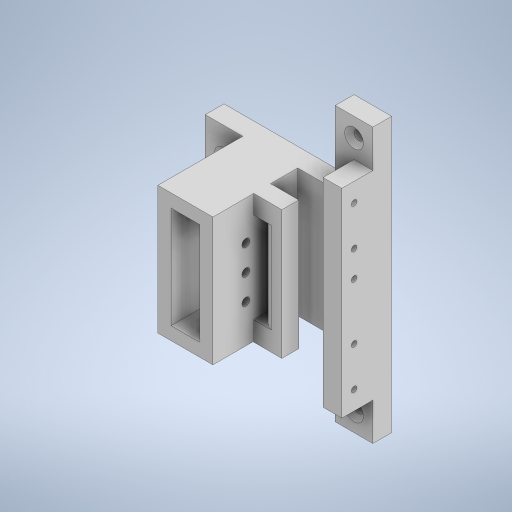
# Autodesk Inventor part: base
Saved by Autodesk Inventor 2024 (Build 280153000, 153)
## iProperties
Created: 2024-06-17
Part Number: base
Material: Generic
Document SubType Name: Modeling
Designer: omiye
Density: 1 g/cm^3
Appearance: Default
Author: omiye
Autodesk Inventor part; units mm, degrees
ref_plane "YZ Plane" through (0, 0, 0) normal (1, 0, 0) x (0, 1, 0)
ref_plane "XZ Plane" through (0, 0, 0) normal (0, 1, 0) x (-1, 0, 0)
ref_plane "XY Plane" through (0, 0, 0) normal (0, 0, 1) x (1, 0, 0)
sketch "Sketch1" plane through (0, 0, 0) normal (1, 0, 0) x (0, 1, 0)
  line L0 (27.1, -22.6) -> (-27.1, -22.6)
  line L1 (-27.1, -22.6) -> (-27.1, 22.6)
  line L2 (-27.1, 22.6) -> (27.1, 22.6)
  line L3 (27.1, 22.6) -> (27.1, -22.6)
  line L4 (27.1, -22.6) -> (-27.1, 22.6) construction
  line L5 (-27.1, -22.6) -> (27.1, 22.6) construction
  point P0 (0, 0)
  dimension "d0" = 54.2
  dimension "d1" = 45.2
  constraints: 12 end point, 2 midpoint, 2 parallel, 1 horizontal, 1 perpendicular
  measures "d0" distance of L1.end L2.end
  measures "d1" distance of L0.end L1.end
extrude "Extrusion1" add sketch "Sketch1" along normal blind 15.3
sketch "Sketch2" plane through (0, 27.1, 22.6) normal (0, 1, 0) x (1, 0, 0)
  line L0 (15.3, 0) -> (15.3, 45.2) projected
  line L1 (0, 0) -> (0, 45.2) projected
  line L2 (15.3, 0) -> (0, 0)
  line L3 (0, 0) -> (0, 45.2)
  line L4 (0, 45.2) -> (15.3, 45.2)
  line L5 (15.3, 45.2) -> (15.3, 0)
  point P0 (0, 22.6)
  constraints: 8 end point, 2 parallel, 1 horizontal, 1 perpendicular
extrude "Extrusion2" add sketch "Sketch2" along normal blind 7
sketch "Sketch3" plane through (0, -27.1, -22.6) normal (0, -1, 0) x (1, 0, 0)
  line L0 (0, 45.2) -> (0, 0) projected
  line L1 (15.3, 45.2) -> (15.3, 0) projected
  line L2 (0, 45.2) -> (15.3, 45.2)
  line L3 (15.3, 45.2) -> (15.3, 0)
  line L4 (15.3, 0) -> (0, 0)
  line L5 (0, 0) -> (0, 45.2)
  point P0 (0, 22.6)
  constraints: 8 end point, 2 parallel, 1 horizontal, 1 perpendicular
extrude "Extrusion3" add sketch "Sketch3" along normal blind 7
sketch "Sketch4" plane through (15.3, 0, 0) normal (1, 0, 0) x (0, 0, -1)
  line L0 (-22.6, -34.1) -> (-22.6, 34.1) projected
  line L1 (-22.6, 34.1) -> (22.6, 34.1) projected
  line L2 (-22.6, -34.1) -> (22.6, -34.1)
  line L3 (22.6, -34.1) -> (22.6, 34.1)
  line L4 (22.6, 34.1) -> (-22.6, 34.1)
  line L5 (-22.6, 34.1) -> (-22.6, -34.1)
  point P0 (0, 0)
  constraints: 8 end point, 2 parallel, 1 horizontal, 1 perpendicular
extrude "Extrusion4" add sketch "Sketch4" along normal blind 7
sketch "Sketch5" plane through (0, 0, 0) normal (-1, 0, 0) x (0, 0, 1)
  line L0 (-22.6, 34.1) -> (22.6, 34.1) projected
  line L1 (22.6, -34.1) -> (-22.6, -34.1) projected
  line L2 (22.6, 34.1) -> (-22.6, 34.1)
  line L3 (-22.6, 34.1) -> (-22.6, -34.1)
  line L4 (-22.6, -34.1) -> (22.6, -34.1)
  line L5 (22.6, -34.1) -> (22.6, 34.1)
  point P0 (0, 0)
  constraints: 8 end point, 2 parallel, 1 horizontal, 1 perpendicular
extrude "Extrusion5" add sketch "Sketch5" along normal blind 7
sketch "Sketch6" plane through (22.3, -34.1, -22.6) normal (0, 0, -1) x (-1, 0, 0)
  line L0 (29.3, 0) -> (0, 0) projected
  line L1 (0, 68.2) -> (0, 0) projected
  line L2 (29.3, 0) -> (0, 0)
  line L3 (0, 0) -> (0, 68.2)
  line L4 (0, 68.2) -> (29.3, 68.2)
  line L5 (29.3, 68.2) -> (29.3, 0)
  point P0 (22.3, 34.1)
  constraints: 8 end point, 2 parallel, 1 horizontal, 1 perpendicular
extrude "Extrusion6" add sketch "Sketch6" along normal blind 10
sketch "Sketch7" plane through (-7, 0, 0) normal (-1, 0, 0) x (0, 0, 1)
  line L0 (22.6, 34.1) -> (-32.6, 34.1) projected
  line L1 (22.6, -34.1) -> (-32.6, -34.1) projected
  line L2 (-32.6, 34.1) -> (-22.6, 34.1)
  line L3 (-22.6, 34.1) -> (-22.6, -34.1)
  line L4 (-22.6, -34.1) -> (-32.6, -34.1)
  line L5 (-32.6, -34.1) -> (-32.6, 34.1)
  point P0 (0, 0)
  dimension "d14" = 10
  constraints: 8 end point, 2 parallel, 1 horizontal, 1 perpendicular, 1 point on line
  measures "d14" distance of L3.end L4.end
extrude "Extrusion7" add sketch "Sketch7" along normal blind 20
sketch "Sketch8" plane through (22.3, -34.1, 22.6) normal (0, 0, 1) x (1, 0, 0)
  line L0 (0, 68.2) -> (-49.3, 68.2) projected
  line L1 (-29.3, 0) -> (-29.3, 68.2) projected
  line L2 (0, 68.2) -> (-29.3, 68.2)
  line L3 (-29.3, 68.2) -> (-29.3, 0)
  line L4 (-29.3, 0) -> (0, 0)
  line L5 (0, 0) -> (0, 68.2)
  line L6 (-22.25, 7) -> (-7.05, 7)
  line L7 (-7.05, 7) -> (-7.05, 61.2)
  line L8 (-7.05, 61.2) -> (-22.25, 61.2)
  line L9 (-22.25, 61.2) -> (-22.25, 7)
  line L10 (-22.25, 7) -> (-7.05, 61.2) construction
  line L11 (-7.05, 7) -> (-22.25, 61.2) construction
  point P0 (-22.3, 34.1)
  point P1 (-14.65, 34.1)
  dimension "d17" = 15.2
  dimension "d18" = 54.2
  constraints: 20 end point, 4 parallel, 2 horizontal, 2 midpoint, 2 perpendicular
  measures "d17" distance of L8.end L7.end
  measures "d18" distance of L7.end L6.end
extrude "Extrusion8" cut sketch "Sketch8" against normal blind 45.2 contours L9 L8 L7 L6
sketch "Sketch9" plane through (22.3, 0, 0) normal (1, 0, 0) x (0, 0, -1)
  line L0 (-22.6, -27.1) -> (22.6, -27.1) projected
  line L1 (-22.6, 27.1) -> (22.6, 27.1) projected
  line L2 (-22.6, -27.1) -> (22.6, -27.1)
  line L3 (22.6, -27.1) -> (22.6, 27.1)
  line L4 (22.6, 27.1) -> (-22.6, 27.1)
  line L5 (-22.6, 27.1) -> (-22.6, -27.1)
  line L6 (-22.6, -27.1) -> (-5.1, -27.1)
  circle A0 centre (-5.1, -13.7) radius 2.1
  circle A1 centre (-5.1, -0.2) radius 2.1
  circle A2 centre (-5.1, 13.4) radius 2.1
  circle A3 centre (12.4, -13.7) radius 2.1
  circle A4 centre (12.4, -0.2) radius 2.1
  circle A5 centre (12.4, 13.4) radius 2.1
  point P0 (0, 0)
  constraints: 10 end point, 6 centre point, 2 parallel, 1 horizontal, 1 perpendicular, 1 point on line
extrude "Extrusion9" cut sketch "Sketch9" against normal blind 39.25 contours A0 | A1 | A2 | A3 | A4 | A5
sketch "Sketch10" plane through (22.3, 0, 0) normal (1, 0, 0) x (0, 0, -1)
  line L0 (-22.6, -34.1) -> (32.6, -34.1) projected
  line L1 (-22.6, 34.1) -> (32.6, 34.1) projected
  line L2 (32.6, -34.1) -> (22.6, -34.1)
  line L3 (22.6, -34.1) -> (22.6, 34.1)
  line L4 (22.6, 34.1) -> (32.6, 34.1)
  line L5 (32.6, 34.1) -> (32.6, -34.1)
  point P0 (0, 0)
  dimension "d36" = 10
  constraints: 8 end point, 2 parallel, 1 horizontal, 1 perpendicular, 1 point on line
  measures "d36" distance of L3.end L4.end
extrude "Extrusion10" add sketch "Sketch10" along normal blind 20
sketch "Sketch11" plane through (42.3, 0, 0) normal (1, 0, 0) x (0, 0, -1)
  line L0 (32.6, 73) -> (22.6, 73)
  line L1 (22.6, 73) -> (22.6, -73)
  line L2 (22.6, -73) -> (32.6, -73)
  line L3 (32.6, -73) -> (32.6, 73)
  line L4 (32.6, 73) -> (22.6, -73) construction
  line L5 (22.6, 73) -> (32.6, -73) construction
  point P0 (0, 0)
  point P1 (27.6, 0)
  dimension "d62" = 10
  dimension "d63" = 146
  constraints: 12 end point, 2 midpoint, 2 parallel, 1 horizontal, 1 perpendicular
  measures "d62" distance of L2.end L1.end
  measures "d63" distance of L1.end L0.end
sketch "Sketch12" plane through (22.3, 0, 0) normal (1, 0, 0) x (0, 0, -1)
  circle A0 centre (-5.1, -0.2) radius 2.1 projected
  circle A1 centre (12.4, -0.2) radius 2.1 projected
  line L0 (-5.1, -0.2) -> (12.4, -0.2)
  line L1 (-22.6, 27.1) -> (22.6, 27.1) projected
  line L2 (-0.85, -27.5) -> (8.15, -27.5)
  line L3 (8.15, -27.5) -> (8.15, 27.1)
  line L4 (8.15, 27.1) -> (-0.85, 27.1)
  line L5 (-0.85, 27.1) -> (-0.85, -27.5)
  line L6 (-0.85, -27.5) -> (8.15, 27.1) construction
  line L7 (8.15, -27.5) -> (-0.85, 27.1) construction
  point P0 (0, 0)
  point P1 (3.65, -0.2)
  dimension "d42" = 9
  constraints: 14 end point, 3 midpoint, 2 horizontal, 2 parallel, 1 perpendicular, 1 point on line
  measures "d42" distance of L4.end L3.end
extrude "Extrusion12" add sketch "Sketch12" along normal blind 15 contours L5 L1 L3 L0 | L0 L3 L2 L5
sketch "Sketch13" plane through (22.3, -27.5, 0.85) normal (0, 0, 1) x (1, 0, 0)
  line L0 (0, 0) -> (15, 0) projected
  line L1 (15, 0) -> (15, 10)
  line L2 (15, 54.6) -> (15, 0) projected
  line L3 (15, 0) -> (25, 0) construction
  line L4 (0, 54.6) -> (15, 54.6) projected
  line L5 (15, 54.6) -> (15, 44.6)
  line L6 (0, 54.6) -> (0, 0) projected
  line L7 (5, 10) -> (5, 44.6)
  line L8 (0, 44.6) -> (0, 10)
  line L9 (0, -6.6) -> (0, 3.4)
  line L10 (0, 61.6) -> (0, 51.6)
  line L11 (0, 61.6) -> (10, 61.6) construction
  line L12 (0, 3.4) -> (5, 3.4)
  line L13 (5, 3.4) -> (5, 51.6)
  line L14 (5, 51.6) -> (0, 51.6)
  line L15 (0, 51.6) -> (0, 3.4)
  point P0 (-22.3, 27.5)
  dimension "d45" = 10
  dimension "d46" = 90
  dimension "d47" = 10
  dimension "d48" = 5
  dimension "d56" = 10
  dimension "d57" = 10
  dimension "d58" = 90
  constraints: 24 end point, 3 horizontal, 3 parallel, 3 perpendicular, 3 point on line, 1 collinear, 1 vertical
  measures "d45" distance of L0.end L1.end
  measures "d46" angle of L3 L1
  measures "d47" distance of L2.start L5.end
  measures "d48" distance of L8.start L7.end
  measures "d56" distance of L9.start L9.end
  measures "d57" distance of L10.start L10.end
  measures "d58" angle of L10 L11
sketch "Sketch14" plane through (22.3, 27.1, 0.85) normal (0, 1, 0) x (1, 0, 0)
  line L0 (15, 9) -> (15, 0) projected
  line L1 (0, 9) -> (0, 0) projected
  line L2 (15, 0) -> (0, 0)
  line L3 (0, 0) -> (0, 9)
  line L4 (0, 9) -> (15, 9)
  line L5 (15, 9) -> (15, 0)
  point P0 (-22.3, 0.85)
  constraints: 8 end point, 2 parallel, 1 horizontal, 1 perpendicular
extrude "Extrusion14" add sketch "Sketch14" along normal blind 7
sketch "Sketch15" plane through (22.3, -27.5, -8.15) normal (0, -1, 0) x (1, 0, 0)
  line L0 (0, 0) -> (0, 9) projected
  line L1 (15, 9) -> (15, 0) projected
  line L2 (0, 9) -> (15, 9)
  line L3 (15, 9) -> (15, 0)
  line L4 (15, 0) -> (0, 0)
  line L5 (0, 0) -> (0, 9)
  point P0 (-22.3, 8.15)
  constraints: 8 end point, 2 parallel, 1 horizontal, 1 perpendicular
extrude "Extrusion15" add sketch "Sketch15" along normal blind 7
extrude "Extrusion16" cut sketch "Sketch13" against normal blind 9.75 contours L6 L14 L13 L7 L12
fillet "Fillet2" radius 4.5 2 edges at (27.3, 0, 0.85) (27.3, 0, -8.15)
extrude "Extrusion17" add sketch "Sketch11" along normal blind 20
sketch "Sketch16" plane through (22.3, -34.1, -22.6) normal (0, 0, 1) x (1, 0, 0)
  line L0 (20, 0) -> (20, -38.9) projected
  line L1 (40, -38.9) -> (40, 107.1) projected
  line L2 (20, -38.9) -> (40, -38.9)
  line L3 (40, -38.9) -> (40, 107.1)
  line L4 (40, 107.1) -> (20, 107.1)
  line L5 (20, 107.1) -> (20, -38.9)
  line L6 (20, -38.9) -> (20, -18.9)
  line L7 (20, -18.9) -> (40, -18.9)
  line L8 (40, -18.9) -> (40, -38.9)
  line L9 (20, 107.1) -> (20, 87.1)
  line L10 (20, 68.2) -> (20, 107.1) projected
  line L11 (20, 87.1) -> (40, 87.1)
  line L12 (40, 107.1) -> (40, 87.1)
  line L13 (40, 107.1) -> (20, 107.1)
  line L14 (40, -18.9) -> (30, -18.9)
  line L15 (30, -18.9) -> (30, 87.1)
  line L16 (30, 87.1) -> (40, 87.1)
  line L17 (40, 87.1) -> (40, -18.9)
  point P0 (-22.3, 34.1)
  dimension "d66" = 20
  dimension "d67" = 20
  dimension "d68" = 10
  constraints: 30 end point, 4 parallel, 4 perpendicular, 4 point on line, 3 collinear, 2 horizontal, 1 midpoint
  measures "d66" distance of L0.end L6.end
  measures "d67" distance of L4.end L9.end
  measures "d68" distance of L15.end L16.end
extrude "Extrusion18" add sketch "Sketch16" along normal blind 20 contours L15 L11 L1 L7
sketch "Sketch17" plane through (62.3, 0, 0) normal (1, 0, 0) x (0, 0, -1)
  line L0 (2.6, -53) -> (2.6, 53) projected
  line L1 (22.6, -53) -> (2.6, -53) projected
  line L2 (2.6, -53) -> (22.6, -53)
  line L3 (22.6, 53) -> (2.6, 53) projected
  line L4 (22.6, -53) -> (22.6, 53)
  line L5 (2.6, 53) -> (2.6, 43)
  line L6 (2.6, 43) -> (2.6, 22)
  line L7 (2.6, -53) -> (2.6, -43)
  line L8 (2.6, -43) -> (2.6, -22)
  line L9 (2.6, 22) -> (2.6, 8)
  line L10 (2.6, -43) -> (12.6, -43)
  circle A0 centre (12.6, -43) radius 1.5
  circle A1 centre (12.6, -22) radius 1.5
  circle A2 centre (12.6, 8) radius 1.5
  circle A3 centre (12.6, 22) radius 1.5
  circle A4 centre (12.6, 43) radius 1.5
  line L11 (2.6, -53) -> (7.6, -53)
  line L12 (7.6, -53) -> (7.6, 53)
  line L13 (7.6, 53) -> (2.6, 53)
  line L14 (2.6, 53) -> (2.6, -53)
  point P0 (0, 0)
  dimension "d71" = 10
  dimension "d72" = 21
  dimension "d73" = 10
  dimension "d74" = 21
  dimension "d75" = 14
  dimension "d76" = 3
  dimension "d77" = 3
  dimension "d78" = 3
  dimension "d79" = 3
  dimension "d80" = 3
  dimension "d81" = 5
  constraints: 24 end point, 6 point on line, 5 centre point, 3 parallel, 2 perpendicular, 1 coincident, 1 collinear, 1 horizontal
  measures "d71" distance of L0.end L5.end
  measures "d72" distance of L5.end L6.end
  measures "d73" distance of L0.start L7.end
  measures "d74" distance of L7.end L8.end
  measures "d75" distance of L6.end L9.end
  measures "d76" diameter of A0
  measures "d77" diameter of A1
  measures "d78" diameter of A2
  measures "d79" diameter of A3
  measures "d80" diameter of A4
  measures "d81" distance of L13.end L12.end
extrude "Extrusion19" cut sketch "Sketch17" against normal blind 20 contours L0 L10 L12 L1 | L0 L3 L12 L10 | A0 | A1 | A2 | A3 | A4
sketch "Sketch18" plane through (62.3, -53, -7.6) normal (0, 0, 1) x (1, 0, 0)
  line L0 (0, 0) -> (-10, 0) projected
  line L1 (0, 106) -> (0, 0) projected
  line L2 (-10, 0) -> (0, 0)
  line L3 (0, 0) -> (0, 106)
  line L4 (0, 106) -> (-10, 106)
  line L5 (-10, 106) -> (-10, 0)
  point P0 (-62.3, 53)
  constraints: 8 end point, 2 parallel, 1 horizontal, 1 perpendicular
extrude "Extrusion20" add sketch "Sketch18" along normal blind 1.5
sketch "Sketch19" plane through (22.3, -34.1, -22.6) normal (0, 0, 1) x (1, 0, 0)
  line L0 (20, 107.1) -> (40, 107.1) projected
  line L1 (30, 107.1) -> (30, 97.1)
  line L2 (20, -38.9) -> (40, -38.9) projected
  line L3 (30, -38.9) -> (30, -28.9)
  line L4 (-29.3, 0) -> (-49.3, 0) projected
  line L5 (-39.3, 0) -> (-39.3, 68.2)
  line L6 (-29.3, 68.2) -> (-49.3, 68.2) projected
  line L7 (-39.3, 68.2) -> (-39.3, 53.2)
  line L8 (-39.3, 0) -> (-39.3, 15)
  line L9 (-39.3, 34.1) -> (-41.2293, 34.1)
  point P0 (-22.3, 34.1)
  dimension "d86" = 10
  dimension "d87" = 10
  dimension "d88" = 15
  dimension "d89" = 15
  constraints: 12 end point, 5 midpoint, 2 point on line, 2 vertical, 1 horizontal
  measures "d86" distance of L1.start L1.end
  measures "d87" distance of L3.start L3.end
  measures "d88" distance of L5.end L7.end
  measures "d89" distance of L5.start L8.end
hole "Hole1" at (-17, 19.1, -22.6) at (-17, 0, -22.6) at (-17, -19.1, -22.6) at (52.3, 63, -22.6) at (52.3, -63, -22.6) direction (0, 0, -1) diameter 5 end through all countersink diameter 10 countersink angle 90
body "Solid1"
